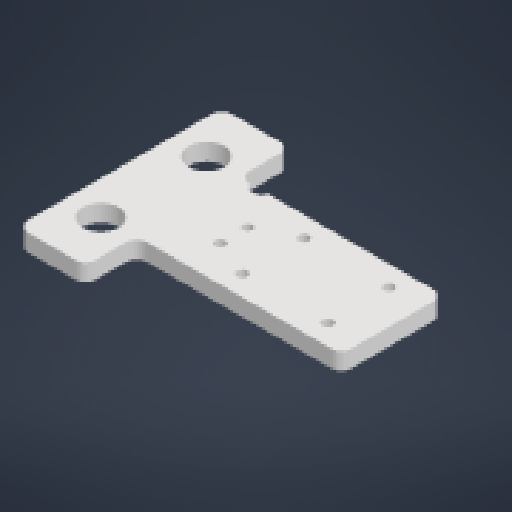
# Autodesk Inventor part: Arm_Top
Saved by Autodesk Inventor 2026.1 (Build 301233020, 233B)
## iProperties
Created: 2025-10-28
Part Number: Arm_Top
Material: Generic
Document SubType Name: Modeling
Designer: Garfieldcmix
Density: 1 g/cm^3
Appearance: Default
Author: Garfieldcmix
Autodesk Inventor part; units mm, degrees
ref_plane "YZ Plane" through (0, 0, 0) normal (1, 0, 0) x (0, 1, 0)
ref_plane "XZ Plane" through (0, 0, 0) normal (0, 1, 0) x (-1, 0, 0)
ref_plane "XY Plane" through (0, 0, 0) normal (0, 0, 1) x (1, 0, 0)
derived "Arm.ipt"
sketch "Sketch1" plane through (0, 0, 0) normal (0, 1, 0) x (-1, 0, 0)
  line L0 (10, 30) -> (10, -30)
  line L1 (10, -30) -> (-10, -30)
  line L2 (-10, -30) -> (-10, -15)
  line L3 (-10, -15) -> (-230, -15)
  line L4 (-230, -15) -> (-230, 15)
  line L5 (-230, 15) -> (-10, 15)
  line L6 (-10, 15) -> (-10, 30)
  line L7 (-10, 30) -> (10, 30)
  line L8 (58, 0) -> (-278, 0) construction
  point P0 (0, 0)
sketch "Sketch2" plane through (0, 8, 0) normal (0, 1, 0) x (1, 0, 0)
  circle A0 centre (0, -15.5) radius 2.9
  circle A1 centre (0, 15.5) radius 2.9
  line L0 (0, 42) -> (0, -42) construction
  line L1 (-58, 0) -> (278, 0) construction
  point P0 (0, 0)
sketch "Sketch3" plane through (0, 8, 0) normal (0, 1, 0) x (1, 0, 0)
  line L0 (230, 15) -> (10, 15) construction
  line L1 (10, -15) -> (230, -15) construction
  line L2 (20, 15) -> (70, 15)
  line L3 (70, 15) -> (70, -15)
  line L4 (70, -15) -> (20, -15)
  line L5 (20, -15) -> (20, 15)
  point P0 (0, 0)
sketch "Sketch4" plane through (0, 13.1, 0) normal (0, 1, 0) x (1, 0, 0)
  circle A0 centre (35, 9) radius 1.475
  circle A1 centre (60, 9) radius 1.475
  circle A2 centre (35, -9) radius 1.475
  circle A3 centre (60, -9) radius 1.475
  line L0 (-58, 0) -> (278, 0) construction
  line L1 (35, 9) -> (35, -9) construction
  line L2 (60, 9) -> (60, -9) construction
  line L3 (20, 15) -> (20, -15) construction
  point P0 (0, 0)
sketch "Sketch5" plane through (0, 0, 0) normal (0, 1, 0) x (-1, 0, 0)
  line L0 (-70, -15) -> (-70, 15) projected
  line L1 (-230, 15) -> (-10, 15) projected
  line L2 (-10, 15) -> (-10, 30) projected
  line L3 (-10, 30) -> (10, 30) projected
  line L4 (10, 30) -> (10, -30) projected
  line L5 (10, -30) -> (-10, -30) projected
  line L6 (-10, -30) -> (-10, -15) projected
  line L7 (-10, -15) -> (-230, -15) projected
  circle A0 centre (-35, 9) radius 1.475 projected
  circle A1 centre (-35, -9) radius 1.475 projected
  circle A2 centre (-60, 9) radius 1.475 projected
  circle A3 centre (-60, -9) radius 1.475 projected
  circle A4 centre (0, 15.5) radius 2.9 construction
  circle A5 centre (0, -15.5) radius 2.9 construction
  circle A6 centre (0, 15.5) radius 5.15
  circle A7 centre (0, -15.5) radius 5.15
  point P0 (0, 0)
  dimension "d3" = 10.3
  constraints: 2 centre point, 2 coincident, 1 equal radius
  measures "d3" diameter of A6
extrude "Extrusion1" add sketch "Sketch5" along normal blind 5
sketch "Sketch6" plane through (0, 5, 0) normal (0, 1, 0) x (1, 0, 0)
  circle A0 centre (0, 15.5) radius 5.15 construction
  line L0 (0, 15.5) -> (16, 15.5) construction
  circle A1 centre (16, 15.5) radius 2.5
  circle A2 centre (24, 3.5) radius 1.45
  circle A3 centre (24, -4.5) radius 1.45
  line L1 (24, 3.5) -> (24, -4.5) construction
  point P0 (0, 0)
  dimension "d4" = 5
  dimension "d5" = 16
  dimension "d8" = 2.9
  dimension "d9" = 24
  dimension "d10" = 8
  dimension "d11" = 12
  constraints: 4 end point, 3 centre point, 1 coincident, 1 equal radius, 1 horizontal, 1 vertical
  measures "d4" diameter of A1
  measures "d5" distance of L0.start L0.end
  measures "d8" diameter of A2
  measures "d9" horizontal distance of L1.start L0.start
  measures "d10" distance of L1.start L1.end
  measures "d11" vertical distance of L1.start L0.start
extrude "Extrusion2" cut sketch "Sketch6" against normal up to surface (5 mm away)
fillet "Fillet1" radius 3 8 edges at (10, 2.5, 15) (10, 2.5, 30) (-10, 2.5, 30) (-10, 2.5, -30) (10, 2.5, -30) (10, 2.5, -15) (70, 2.5, 15) (70, 2.5, -15)
body "Solid1"
